001 (Autodesk Fusion 360 design; units mm, degrees)
Autodesk Fusion 360 part; units mm, degrees
sketch "Esquisse1" plane through (0, 0, 0) normal (0, 0, 1) x (1, 0, 0)
  line L0 (-75, 95) -> (75, 95)
  line L1 (75, 95) -> (75, -60)
  line L2 (75, -60) -> (-75, -60)
  line L3 (-75, -60) -> (-75, 95)
  line L4 (0, 1.75) -> (0, 22.5)
  line L5 (1.75, 0) -> (22.5, 0)
  line L6 (20, 0) -> (2.5, 0)
  dimension "d1" = 150
  dimension "d2" = 155
  dimension "d69" = 95
  constraint horizontal L0
  constraint vertical L1
  constraint horizontal L2
  constraint vertical L3
  constraint symmetric L1 L3 L4
  measures "d1" distance of L0.start L0.end
  measures "d2" distance of L0.start L2.end
  measures "d69" distance of L0 L6
extrude "Extrusion1" add sketch "Esquisse1" against normal blind 25
sketch "Esquisse2" plane through (0, 0, 0) normal (0, 0, 1) x (-1, 0, 0)
  line L0 (75, 60) -> (-75, 60)
  line L1 (-75, 60) -> (-75, -95)
  line L2 (-75, -95) -> (75, -95)
  line L3 (75, -95) -> (75, 60)
  circle A0 centre (0, 0) radius 11.125
  dimension "d5" = 22.25
  constraint coincident A0.centre origin
  measures "d5" diameter of A0
extrude "Extrusion2" cut sketch "Esquisse2" against normal blind 12 contours A0
sketch "Esquisse3" plane through (0, 0, -25) normal (0, 0, -1) x (1, 0, 0)
  line L0 (75, 60) -> (-75, 60)
  line L1 (-75, 60) -> (-75, -95)
  line L2 (-75, -95) -> (75, -95)
  line L3 (75, -95) -> (75, 60)
sketch "Esquisse4" plane through (0, 0, -25) normal (0, 0, -1) x (1, 0, 0)
  circle A0 centre (0, 0) radius 11.125
  dimension "d8" = 22.25
  constraint coincident A0.centre origin
  measures "d8" diameter of A0
extrude "Extrusion3" cut sketch "Esquisse4" against normal blind 10
sketch "Esquisse5" plane through (0, 0, -12) normal (0, 0, 1) x (-1, 0, 0)
  circle A0 centre (0, 0) radius 11.125
  circle A1 centre (0, 0) radius 4
  dimension "d11" = 8
  constraint concentric A0 A1
  measures "d11" diameter of A1
extrude "Extrusion4" cut sketch "Esquisse5" against normal blind 51 contours A1
sketch "Esquisse6" plane through (0, 0, 0) normal (0, 0, 1) x (-1, 0, 0)
  circle A0 centre (0, 0) radius 11.125
  line L0 (75, 60) -> (-75, 60)
  line L1 (-75, 60) -> (-75, -95)
  line L2 (-75, -95) -> (75, -95)
  line L3 (75, -95) -> (75, 60)
  line L4 (-21.1, -45) -> (21.1, -45)
  line L5 (21.1, -45) -> (21.1, -87.2)
  line L6 (21.1, -87.2) -> (-21.1, -87.2)
  line L7 (-21.1, -87.2) -> (-21.1, -45)
  line L8 (-20, 0) -> (-2.5, 0)
  line L9 (0, -1.75) -> (0, -22.5)
  dimension "d14" = 45
  dimension "d15" = 42.2
  dimension "d16" = 42.2
  constraint horizontal L4
  constraint vertical L5
  constraint horizontal L6
  constraint vertical L7
  constraint symmetric L5 L7 L9
  measures "d14" distance of L4 L8
  measures "d15" distance of L4.start L4.end
  measures "d16" distance of L4.start L6.end
extrude "Extrusion5" cut sketch "Esquisse6" against normal blind 17 contours L4 L5 L6 L7
fillet "Congé1" radius 3 4 edges at (21.1, 87.2, -8.5) (21.1, 45, -8.5) (-21.1, 87.2, -8.5) (-21.1, 45, -8.5)
sketch "Esquisse7" plane through (0, 0, -17) normal (0, 0, 1) x (-1, 0, 0)
  arc A0 (21.1, -48) -> (18.1, -45) centre (18.1, -48) ccw
  line L0 (18.1, -45) -> (-18.1, -45)
  arc A1 (-18.1, -45) -> (-21.1, -48) centre (-18.1, -48) ccw
  line L1 (-21.1, -48) -> (-21.1, -84.2)
  line L2 (21.1, -84.2) -> (21.1, -48)
  circle A2 centre (0, -66.1) radius 11.1
  line L3 (21.1, -48) -> (21.1, -84.2)
  line L4 (18.1, -87.2) -> (-18.1, -87.2)
  arc A3 (-21.1, -84.2) -> (-18.1, -87.2) centre (-18.1, -84.2) ccw
  line L5 (-18.1, -87.2) -> (18.1, -87.2)
  arc A4 (18.1, -87.2) -> (21.1, -84.2) centre (18.1, -84.2) ccw
  dimension "d21" = 22.2
  dimension "d22" = 21.1
  dimension "d23" = 21.1
  measures "d21" diameter of A2
  measures "d22" distance of A2.centre L3
  measures "d23" distance of A2.centre L4
extrude "Extrusion6" cut sketch "Esquisse7" against normal blind 2.5 contours A2
sketch "Esquisse8" plane through (0, 0, -19.5) normal (0, 0, 1) x (-1, 0, 0)
  circle A0 centre (0, -66.1) radius 3
  circle A1 centre (0, -66.1) radius 11.1
  circle A2 centre (0, -66.1) radius 11.1
  dimension "d26" = 6
  constraint concentric A0 A2
  measures "d26" diameter of A0
extrude "Extrusion7" cut sketch "Esquisse8" against normal blind 33 contours A0
sketch "Esquisse9" plane through (0, 0, -17) normal (0, 0, 1) x (-1, 0, 0)
  arc A0 (21.1, -48) -> (18.1, -45) centre (18.1, -48) ccw
  line L0 (18.1, -45) -> (-18.1, -45)
  arc A1 (-18.1, -45) -> (-21.1, -48) centre (-18.1, -48) ccw
  line L1 (-21.1, -48) -> (-21.1, -84.2)
  line L2 (21.1, -84.2) -> (21.1, -48)
  circle A2 centre (0, -66.1) radius 11.1
  arc A3 (-21.1, -84.2) -> (-18.1, -87.2) centre (-18.1, -84.2) ccw
  line L3 (-18.1, -87.2) -> (18.1, -87.2)
  arc A4 (18.1, -87.2) -> (21.1, -84.2) centre (18.1, -84.2) ccw
  point P0 (-15.5, -50.6)
  point P1 (15.5, -50.6)
  point P2 (-15.5, -81.6)
  point P3 (15.5, -81.6)
  dimension "d29" = 15.5
  dimension "d30" = 15.5
  dimension "d33" = 31
  dimension "d34" = -31
  measures "d29" vertical distance of P0 A2.centre
  measures "d30" horizontal distance of P0 A2.centre
hole "Perçage1" at (15.5, 50.6, -17) at (-15.5, 50.6, -17) at (-15.5, 81.6, -17) at (15.5, 81.6, -17) direction (0, 0, -1) diameter 4 depth 30 tip angle 118
mirror "Symétrie miroir1" [suppressed]
sketch "Esquisse10" plane through (0, 0, -25) normal (0, 0, -1) x (1, 0, 0)
  line L0 (1.75, 0) -> (22.5, 0)
  line L1 (0, -1.75) -> (0, -22.5)
  line L2 (0, -2.5) -> (0, -20)
  line L3 (20, 0) -> (2.5, 0)
  line L4 (-75, -95) -> (75, -95)
  line L5 (-75, 60) -> (-75, -95)
  point P0 (-63, -83)
  dimension "d74" = 12
  dimension "d75" = 12
  measures "d74" distance of P0 L4
  measures "d75" distance of P0 L5
hole "Perçage2" at (-63, 83, -25) direction (0, 0, 1) diameter 5 depth 30 tip angle 118
sketch "Esquisse11" plane through (-75, 0, 0) normal (-1, 0, 0) x (0, -1, 0)
  line L0 (60, 0) -> (-95, 0)
  line L1 (-95, 0) -> (-95, -25)
  line L2 (-95, -25) -> (60, -25)
  line L3 (60, -25) -> (60, 0)
  circle A0 centre (-35, -12.5) radius 4.125
  line L4 (60, -25) -> (-95, -25)
  line L5 (0, 2.5) -> (0, 20)
  dimension "d49" = 8.25
  dimension "d50" = 12.5
  dimension "d51" = 35
  measures "d49" diameter of A0
  measures "d50" distance of A0.centre L4
  measures "d51" distance of A0.centre L5
extrude "Extrusion8" cut sketch "Esquisse11" against normal blind 165 contours A0
mirror "Symétrie miroir2" about plane through (0, 0, 0) normal (0, 1, 0) of "Extrusion8"
sketch "Esquisse12" plane through (0, 0, -25) normal (0, 0, -1) x (1, 0, 0)
sketch "Esquisse13" plane through (0, 0, -25) normal (0, 0, -1) x (1, 0, 0)
sketch "Esquisse14" plane through (0, 0, -25) normal (0, 0, -1) x (1, 0, 0)
  arc A0 (55, 19.2) -> (55, 15) centre (55, 17.1) ccw
  line L0 (55, 19.2) -> (63, 19.2)
  arc A1 (63, 15) -> (63, 19.2) centre (63, 17.1) ccw
  line L1 (55, 15) -> (63, 15)
  line L2 (0, -1.75) -> (0, -22.5)
  line L3 (1.75, 0) -> (22.5, 0)
  line L4 (0, -2.5) -> (0, -20)
  dimension "d57" = 8
  dimension "d60" = 4.2
  dimension "d70" = 15
  dimension "d71" = 55
  constraint tangent A0 L0
  constraint tangent L0 A1
  constraint tangent A0 L1
  constraint tangent A1 L1
  constraint parallel L0 L1
  measures "d57" distance of A0.start L0.end
  measures "d60" distance of L0 L1
  measures "d70" distance of L1 L3
  measures "d71" distance of A0.end L4
extrude "Extrusion9" cut sketch "Esquisse14" against normal blind 35
pattern_linear "Réseau R1" count 2 spacing 31 along (0, -1, 0) count 2 spacing 31 along (-1, 0, 0) of "Extrusion9"
sketch "Esquisse15" plane through (0, 0, 0) normal (0, 0, 1) x (-1, 0, 0)
  line L0 (-24, 46) -> (-32, 46)
  arc A0 (-32, 50.2) -> (-32, 46) centre (-32, 48.1) ccw
  line L1 (-32, 50.2) -> (-24, 50.2)
  arc A1 (-24, 46) -> (-24, 50.2) centre (-24, 48.1) ccw
  line L2 (-24, 15) -> (-32, 15)
  arc A2 (-32, 19.2) -> (-32, 15) centre (-32, 17.1) ccw
  line L3 (-32, 19.2) -> (-24, 19.2)
  arc A3 (-24, 15) -> (-24, 19.2) centre (-24, 17.1) ccw
  line L4 (-55, 46) -> (-63, 46)
  arc A4 (-63, 50.2) -> (-63, 46) centre (-63, 48.1) ccw
  line L5 (-63, 50.2) -> (-55, 50.2)
  arc A5 (-55, 46) -> (-55, 50.2) centre (-55, 48.1) ccw
  line L6 (-55, 15) -> (-63, 15)
  arc A6 (-63, 19.2) -> (-63, 15) centre (-63, 17.1) ccw
  line L7 (-63, 19.2) -> (-55, 19.2)
  arc A7 (-55, 15) -> (-55, 19.2) centre (-55, 17.1) ccw
  circle A8 centre (63, -83) radius 2.5
  line L8 (21.1, -48) -> (21.1, -84.2)
  arc A9 (18.1, -87.2) -> (21.1, -84.2) centre (18.1, -84.2) ccw
  line L9 (18.1, -87.2) -> (-18.1, -87.2)
  arc A10 (-21.1, -84.2) -> (-18.1, -87.2) centre (-18.1, -84.2) ccw
  line L10 (-21.1, -84.2) -> (-21.1, -48)
  arc A11 (-18.1, -45) -> (-21.1, -48) centre (-18.1, -48) ccw
  line L11 (-18.1, -45) -> (18.1, -45)
  arc A12 (21.1, -48) -> (18.1, -45) centre (18.1, -48) ccw
  circle A13 centre (0, 0) radius 11.125
  line L12 (75, 60) -> (-75, 60)
  line L13 (-75, 60) -> (-75, -95)
  line L14 (-75, -95) -> (75, -95)
  line L15 (75, -95) -> (75, 60)
  point P0 (63, 48)
  dimension "d76" = 12
  dimension "d77" = 12
  measures "d76" distance of L12 P0
  measures "d77" distance of L15 P0
hole "Perçage3" at (-63, -48, 0) direction (0, 0, -1) diameter 5 depth 50 tip angle 118
fillet "Congé2" radius 10 1 edges at (-75, 95, -12.5)
fillet "Congé2" radius 10 3 edges at (75, 95, -12.5) (75, -60, -12.5) (-75, -60, -12.5)
sketch "Esquisse16" plane through (0, 0, -25) normal (0, 0, -1) x (1, 0, 0)
sketch "Esquisse17" plane through (0, 0, -25) normal (0, 0, -1) x (1, 0, 0)
  circle A0 centre (-63, 48) radius 10.25
  line L0 (75, 60) -> (-75, 60)
  line L1 (-75, 60) -> (-75, -95)
  dimension "d85" = 20.5
  dimension "d86" = 12
  dimension "d87" = 12
  measures "d85" diameter of A0
  measures "d86" distance of A0.centre L0
  measures "d87" distance of A0.centre L1
extrude "Extrusion10" cut sketch "Esquisse17" against normal blind 1
sketch "Esquisse18" plane through (0, 0, -25) normal (0, 0, -1) x (1, 0, 0)
  circle A0 centre (-63, -83) radius 10.25
  line L0 (-75, 60) -> (-75, -95)
  line L1 (-75, -95) -> (75, -95)
  dimension "d90" = 20.5
  dimension "d91" = 12
  dimension "d92" = 12
  measures "d90" diameter of A0
  measures "d91" distance of A0.centre L0
  measures "d92" distance of A0.centre L1
extrude "Extrusion11" cut sketch "Esquisse18" against normal blind 1
equation "d22 = ( 42.2 / 2 ) * 1 mm"
equation "d23 = ( 42.2 / 2 ) * 1 mm"
equation "d29 = ( 31 / 2 ) * 1 mm"
equation "d30 = ( 31 / 2 ) * 1 mm"
equation "d50 = ( 25 / 2 ) * 1 mm"
